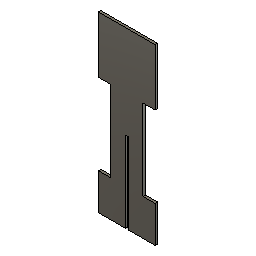
Creeper - Montagem (Autodesk Fusion 360 archive; units mm, degrees)
design "1"
Autodesk Fusion 360 part; units mm, degrees
sketch "Sketch1" plane through (0, 0, 0) normal (0, 0, 1) x (1, 0, 0)
  line L0 (0, 0) -> (70, 0)
  line L1 (70, 0) -> (70, 70)
  line L2 (70, 70) -> (0, 70)
  line L3 (0, 70) -> (0, 0)
  line L4 (70, 0) -> (55, 0)
  line L5 (0, 0) -> (15, 0)
  line L6 (15, 0) -> (15, -100)
  line L7 (55, 0) -> (55, -100)
  line L8 (55, -100) -> (70, -100)
  line L9 (15, -100) -> (0, -100)
  line L10 (0, -100) -> (0, -145)
  line L11 (70, -100) -> (70, -145)
  line L12 (70, -145) -> (0, -145)
  line L13 (35, -145) -> (36.55, -145)
  line L14 (35, -145) -> (33.45, -145)
  line L15 (36.55, -145) -> (36.55, -45)
  line L16 (33.45, -145) -> (33.45, -45)
  line L17 (33.45, -45) -> (36.55, -45)
  dimension "d1" = 70
  dimension "d2" = 70
  dimension "d3" = 15
  dimension "d4" = 15
  dimension "d5" = 100
  dimension "d6" = 100
  dimension "d7" = 15
  dimension "d8" = 15
  dimension "d9" = 45
  dimension "d10" = 45
  dimension "d11" = 1.55
  dimension "d12" = 1.55
  dimension "d13" = 100
  dimension "d14" = 100
  dimension "d17" = 33.25
  dimension "d18" = 33.25
  constraint horizontal L0
  constraint vertical L1
  constraint horizontal L2
  constraint vertical L3
  constraint coincident L0.start L3.end
  constraint perpendicular L1 L4
  constraint perpendicular L3 L5
  constraint perpendicular L0 L6
  constraint perpendicular L4 L7
  constraint perpendicular L7 L8
  constraint perpendicular L6 L9
  constraint perpendicular L9 L10
  constraint perpendicular L8 L11
  constraint midpoint L12 L13.start
  constraint horizontal L13
  constraint parallel L12 L14
  constraint perpendicular L13 L15
  constraint perpendicular L12 L16
  measures "d1" distance of L0.start L0.end
  measures "d2" distance of L0.start L2.end
  measures "d3" distance of L0.end L4.end
  measures "d4" distance of L0.start L5.end
  measures "d5" distance of L5.end L6.end
  measures "d6" distance of L4.end L7.end
  measures "d7" distance of L7.end L8.end
  measures "d8" distance of L6.end L9.end
  measures "d9" distance of L9.end L10.end
  measures "d10" distance of L8.end L11.end
  measures "d11" distance of L13.start L13.end
  measures "d12" distance of L13.start L14.end
  measures "d13" distance of L13.end L15.end
  measures "d14" distance of L14.end L16.end
extrude "Extrude1" add sketch "Sketch1" along normal blind 3 contours L0 L1 L2 L3 L4 L5 | L0 L6 L7 L8 L9 L10 L11 L12 L15 L16 L17
